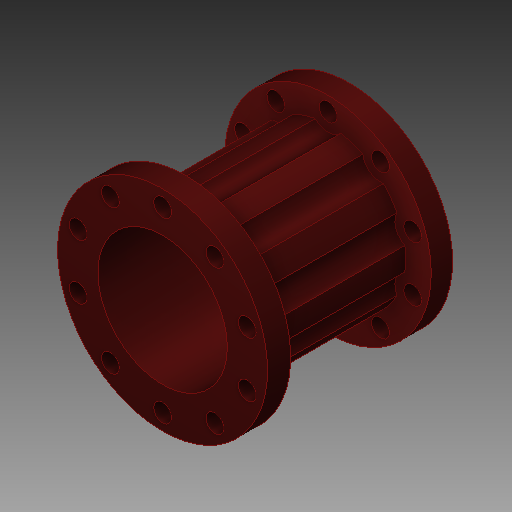
# Autodesk Inventor part: 212-01
Saved by Autodesk Inventor 2019 (Build 230136000, 136)
## iProperties
Company: Autodesk Inc.
Created: 2017-03-14
Part Number: 212-01
Material: Titanium
Document SubType Name: Modeling
Designer: Autodesk Inc.
Density: 4.51 g/cm^3
Appearance: Anodized - Dark Red
Mass: 148.417 g
Surface Area: 211.033 cm^2
Volume: 32.9085 cm^3
Author: Inventor
Autodesk Inventor part; units mm, degrees
ref_plane "YZ Plane" through (0, 0, 0) normal (1, 0, 0) x (0, 1, 0)
ref_plane "XZ Plane" through (0, 0, 0) normal (0, 1, 0) x (-1, 0, 0)
ref_plane "XY Plane" through (0, 0, 0) normal (0, 0, 1) x (1, 0, 0)
sketch "Sketch1" plane through (0, 0, 0) normal (0, 0, 1) x (1, 0, 0)
  circle A0 centre (0, 0) radius 21.823
  circle A1 centre (0, 0) radius 18.188
  dimension "d1" = 43.646
  dimension "d2" = 36.376
  constraints: 2 centre point, 2 coincident
  measures "d1" diameter of A0
  measures "d2" diameter of A1
extrude "Extrusion1" add sketch "Sketch1" along normal blind 40
sketch "Sketch2" plane through (0, 0, 40) normal (0, 0, 1) x (1, 0, 0)
  circle A0 centre (0, 0) radius 18.188 projected
  circle A1 centre (0, 0) radius 21.823 projected
  circle A2 centre (0, 0) radius 29.5
  dimension "d5" = 59
  constraints: 1 centre point, 1 coincident
  measures "d5" diameter of A2
extrude "Extrusion2" add sketch "Sketch2" along normal blind 6.5 contours A1 | A2
sketch "Sketch3" plane through (0, 0, 0) normal (0, 0, -1) x (-1, 0, 0)
  circle A0 centre (0, 0) radius 18.188 projected
  circle A1 centre (0, 0) radius 21.823 projected
  circle A2 centre (0, 0) radius 29
  dimension "d8" = 58
  constraints: 1 centre point, 1 coincident
  measures "d8" diameter of A2
extrude "Extrusion3" add sketch "Sketch3" along normal blind 6 contours A1 | A2
fillet "Fillet1" radius 2 1 edges at (-21.823, 0, 40)
sketch "Sketch4" plane through (0, 0, 46.5) normal (0, 0, 1) x (1, 0, 0)
  circle A0 centre (0, 0) radius 18.188 projected
  point P0 (0, 25)
  dimension "d12" = 25
  constraints: 1 vertical alignment
  measures "d12" distance of A0.centre point (0, 25)
hole "Hole1" at (0, 25, 46.5) direction (0, 0, -1) diameter 5 end through all
pattern_circular "Circular Pattern1" count 10 over 360 about axis through (0, 0, -10) along (0, 0, 1) of "Hole1"
sketch "Sketch6" plane through (0, 0, 0) normal (1, 0, 0) x (0, 1, 0)
  line L0 (-27.5, 0) -> (-27.5, -6) projected
  line L1 (-27.5, -6) -> (-29, -6) projected
  line L2 (-29, -6) -> (-29, 0) projected
  line L3 (-29, 0) -> (-27.5, 0) projected
  line L4 (-27.5, 46.5) -> (-27.5, 40) projected
  line L5 (-27.5, 40) -> (-29.5, 40) projected
  line L6 (-29.5, 40) -> (-29.5, 46.5) projected
  line L7 (-29.5, 46.5) -> (-27.5, 46.5) projected
  line L8 (-22.5, 39.4999) -> (-22.5, 46.5) projected
  line L9 (-22.5, 46.5) -> (-18.188, 46.5) projected
  line L10 (-18.188, 46.5) -> (-18.188, -6) projected
  line L11 (-18.188, -6) -> (-22.5, -6) projected
  line L12 (-22.5, -6) -> (-22.5, 0) projected
  line L13 (-22.5, 0) -> (-21.823, 0) projected
  line L14 (-21.823, 0) -> (-21.823, 38) projected
  arc A0 (-21.823, 38) -> (-22.5, 39.4999) centre (-23.823, 38) ccw projected
  line L15 (29.5, 40) -> (27.5, 40) projected
  line L16 (27.5, 40) -> (27.5, 46.5) projected
  line L17 (27.5, 46.5) -> (29.5, 46.5) projected
  line L18 (29.5, 46.5) -> (29.5, 40) projected
  line L19 (27.5, -6) -> (27.5, 0) projected
  line L20 (27.5, 0) -> (29, 0) projected
  line L21 (29, 0) -> (29, -6) projected
  line L22 (29, -6) -> (27.5, -6) projected
  line L23 (22.5, 0) -> (22.5, -6) projected
  line L24 (22.5, -6) -> (18.188, -6) projected
  line L25 (18.188, -6) -> (18.188, 46.5) projected
  line L26 (18.188, 46.5) -> (22.5, 46.5) projected
  line L27 (22.5, 46.5) -> (22.5, 39.4999) projected
  arc A1 (22.5, 39.4999) -> (21.823, 38) centre (23.823, 38) ccw projected
  line L28 (21.823, 38) -> (21.823, 0) projected
  line L29 (21.823, 0) -> (22.5, 0) projected
  line L30 (25, 50.0408) -> (25, 14.0818)
  line L31 (25, 40) -> (30, 40)
  line L32 (30, 40) -> (30, 0)
  line L33 (30, 0) -> (25, 0)
  line L34 (25, 40) -> (25, 0)
  point P0 (29, 0)
  dimension "d27" = 5
  dimension "d28" = 5
  dimension "d29" = 40
  constraints: 10 end point, 4 point on line, 2 collinear, 2 perpendicular, 1 vertical
  measures "d27" diameter of L16 L30
  measures "d28" distance of L31.start L31.end
  measures "d29" distance of L32.end L31.end
revolve "Revolution1" cut sketch "Sketch6" angle 360 about axis through (0, 25, 50.0408) along (0, 0, -1) contours L31 L32 L33 L20 L34 L30 L15
pattern_circular "Circular Pattern2" count 10 over 360 about axis through (0, 0, -10) along (0, 0, 1) of "Revolution1"
body "Solid1"
